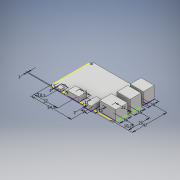
# Autodesk Inventor part: RasPi3B+
Saved by Autodesk Inventor 2017 (Build 210142000, 142)
## iProperties
Part Number: RasPi3B+
Material: Genérico
Document SubType Name: Modeling
Designer: danie
Density: 1 g/cm^3
Appearance: Valor por defecto
Author: danie
Autodesk Inventor part; units mm, degrees
ref_plane "YZ Plane" through (0, 0, 0) normal (1, 0, 0) x (0, 1, 0)
ref_plane "XZ Plane" through (0, 0, 0) normal (0, 1, 0) x (-1, 0, 0)
ref_plane "XY Plane" through (0, 0, 0) normal (0, 0, 1) x (1, 0, 0)
sketch "Boceto1" plane through (0, 0, 0) normal (0, 0, 1) x (1, 0, 0)
  line L0 (-39.5, -28) -> (39.5, -28)
  line L1 (42.5, -25) -> (42.5, 25)
  line L2 (39.5, 28) -> (-39.5, 28)
  line L3 (-42.5, 25) -> (-42.5, -25)
  line L4 (-42.5, -28) -> (42.5, 28) construction
  line L5 (42.5, -28) -> (-42.5, 28) construction
  arc A0 (-39.5, 28) -> (-42.5, 25) centre (-39.5, 25) ccw
  arc A1 (42.5, 25) -> (39.5, 28) centre (39.5, 25) ccw
  arc A2 (39.5, -28) -> (42.5, -25) centre (39.5, -25) ccw
  arc A3 (-42.5, -25) -> (-39.5, -28) centre (-39.5, -25) ccw
  circle A4 centre (-39.5, 25) radius 1.375
  circle A5 centre (-39.5, -25) radius 1.375
  circle A6 centre (18.5, -25) radius 1.375
  circle A7 centre (18.5, 25) radius 1.375
  point P0 (0, 0)
  dimension "d0" = 85
  dimension "d1" = 56
  dimension "d2" = 3
  dimension "d3" = 2.75
  dimension "d4" = 2.75
  dimension "d5" = 2.75
  dimension "d6" = 2.75
  dimension "d7" = 58
  constraints: 12 end point, 8 centre point, 8 point on circle, 8 point on line, 8 tangent, 3 equal radius, 2 coincident, 2 horizontal alignment, 2 midpoint, 2 parallel, 1 horizontal, 1 perpendicular, 1 vertical alignment
  measures "d0" distance of L5.end L4.end
  measures "d1" distance of L4.end L5.start
  measures "d2" radius of A0
  measures "d3" diameter of A4
  measures "d4" diameter of A5
  measures "d5" diameter of A6
  measures "d6" diameter of A7
  measures "d7" distance of A7.centre A0.centre
extrude "Extrusión1" add sketch "Boceto1" along normal blind 2
sketch "Boceto2" plane through (0, 0, 2) normal (0, 0, 1) x (1, 0, 0)
  line L0 (26.5, -6.5) -> (44.5, -6.5)
  line L1 (44.5, -6.5) -> (44.5, 8.5)
  line L2 (44.5, 8.5) -> (26.5, 8.5)
  line L3 (26.5, 8.5) -> (26.5, -6.5)
  line L4 (26.5, -6.5) -> (44.5, 8.5) construction
  line L5 (44.5, -6.5) -> (26.5, 8.5) construction
  line L6 (-39.5, -28) -> (39.5, -28) projected
  line L7 (22.5, -25.75) -> (44.5, -25.75)
  line L8 (44.5, -25.75) -> (44.5, -9.75)
  line L9 (44.5, -9.75) -> (22.5, -9.75)
  line L10 (22.5, -9.75) -> (22.5, -25.75)
  line L11 (22.5, -25.75) -> (44.5, -9.75) construction
  line L12 (44.5, -25.75) -> (22.5, -9.75) construction
  line L13 (-18, -29) -> (-3, -29)
  line L14 (-3, -29) -> (-3, -18)
  line L15 (-3, -18) -> (-18, -18)
  line L16 (-18, -18) -> (-18, -29)
  line L17 (-18, -29) -> (-3, -18) construction
  line L18 (-3, -29) -> (-18, -18) construction
  line L19 (-42.5, 25) -> (-42.5, -25) projected
  line L20 (8, -16) -> (16, -16)
  line L21 (16, -16) -> (16, -31)
  line L22 (16, -31) -> (8, -31)
  line L23 (8, -31) -> (8, -16)
  line L24 (8, -16) -> (16, -31) construction
  line L25 (16, -16) -> (8, -31) construction
  line L26 (-36.5, -29) -> (-27.5, -29)
  line L27 (-27.5, -29) -> (-27.5, -24)
  line L28 (-27.5, -24) -> (-36.5, -24)
  line L29 (-36.5, -24) -> (-36.5, -29)
  line L30 (-36.5, -29) -> (-27.5, -24) construction
  line L31 (-27.5, -29) -> (-36.5, -24) construction
  line L32 (26.5, 11.5) -> (44.5, 11.5)
  line L33 (44.5, 11.5) -> (44.5, 26.5)
  line L34 (44.5, 26.5) -> (26.5, 26.5)
  line L35 (26.5, 26.5) -> (26.5, 11.5)
  line L36 (26.5, 11.5) -> (44.5, 26.5) construction
  line L37 (44.5, 11.5) -> (26.5, 26.5) construction
  line L38 (42.5, -25) -> (42.5, 25) projected
  point P0 (0, 0)
  point P1 (35.5, 1)
  point P2 (33.5, -17.75)
  point P3 (-10.5, -23.5)
  point P4 (12, -23.5)
  point P5 (-32, -26.5)
  point P6 (35.5, 19)
  dimension "d11" = 15
  dimension "d15" = 29
  dimension "d18" = 22
  dimension "d19" = 16
  dimension "d20" = 10.25
  dimension "d22" = 15
  dimension "d23" = 11
  dimension "d24" = 1
  dimension "d25" = 32
  dimension "d26" = 8
  dimension "d27" = 15
  dimension "d28" = 3
  dimension "d29" = 54.5
  dimension "d30" = 9
  dimension "d31" = 5
  dimension "d33" = 1
  dimension "d34" = 10.5
  dimension "d45" = 15
  dimension "d46" = 2
  dimension "d47" = 47
  constraints: 72 end point, 12 midpoint, 12 parallel, 6 horizontal, 6 perpendicular
  measures "d11" distance of L1.end L0.end
  measures "d15" distance from line of L6 point (35.5, 1)
  measures "d18" distance of L9.end L8.end
  measures "d19" distance of L8.end L7.end
  measures "d20" distance from line of L6 point (33.5, -17.75)
  measures "d22" distance of L15.end L14.end
  measures "d23" distance of L14.end L13.end
  measures "d24" distance between parallel lines of L6 L13
  measures "d25" distance from line of L19 point (-10.5, -23.5)
  measures "d26" distance of L21.end L22.end
  measures "d27" distance of L20.end L21.end
  measures "d28" distance between parallel lines of L6 L22
  measures "d29" distance from line of L19 point (12, -23.5)
  measures "d30" distance of L28.end L27.end
  measures "d31" distance of L27.end L26.end
  measures "d33" distance between parallel lines of L6 L26
  measures "d34" distance from line of L19 point (-32, -26.5)
  measures "d45" distance of L33.end L32.end
  measures "d46" distance between parallel lines of L33 L38
  measures "d47" distance from line of L6 point (35.5, 19)
extrude "Extrusión3" add sketch "Boceto2" along normal blind 13.5 contours L9 L8 L7 L10
extrude "Extrusión4" add sketch "Boceto2" along normal blind 6 contours L23 L20 L21 L6 | L6 L21 L22 L23
extrude "Extrusión5" add sketch "Boceto2" along normal blind 6.5 contours L16 L15 L14 L6 | L6 L14 L13 L16
extrude "Extrusión6" add sketch "Boceto2" along normal blind 3 contours L29 L28 L27 L6 | L6 L27 L26 L29
extrude "Extrusión7" add sketch "Boceto2" along normal blind 16 contours L3 L2 L38 L0 | L32 L35 L34 L33 | L38 L2 L1 L0
